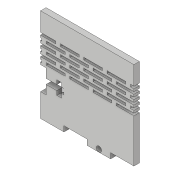
# Autodesk Inventor part: side2+hinge
Saved by Autodesk Inventor 2017 (Build 210142000, 142)
## iProperties
Created: 2019-05-21
Part Number: side2+hinge
Material: Generic
Document SubType Name: Modeling
Designer: markg
Density: 1 g/cm^3
Appearance: Default
Author: markg
Autodesk Inventor part; units mm, degrees
ref_plane "YZ Plane" through (0, 0, 0) normal (1, 0, 0) x (0, 1, 0)
ref_plane "XZ Plane" through (0, 0, 0) normal (0, 1, 0) x (-1, 0, 0)
ref_plane "XY Plane" through (0, 0, 0) normal (0, 0, 1) x (1, 0, 0)
sketch "Sketch1" plane through (0, 0, 0) normal (0, 0, 1) x (1, 0, 0)
  line L0 (-25.4, -25.4) -> (25.4, -25.4)
  line L1 (25.4, -25.4) -> (25.4, 25.4)
  line L2 (25.4, 25.4) -> (-25.4, 25.4)
  line L3 (-25.4, 25.4) -> (-25.4, -25.4)
  line L4 (-25.4, -25.4) -> (25.4, 25.4) construction
  line L5 (25.4, -25.4) -> (-25.4, 25.4) construction
  point P0 (0, 0)
  dimension "d0" = 50.8
  dimension "d1" = 50.8
  constraints: 12 end point, 2 midpoint, 2 parallel, 1 horizontal, 1 perpendicular
  measures "d0" distance of L2.end L1.end
  measures "d1" distance of L1.end L0.end
extrude "Extrusion1" add sketch "Sketch1" along normal blind 2.9718
sketch "Sketch2" plane through (0, 0, 2.9718) normal (0, 0, 1) x (1, 0, 0)
  line L0 (-25.4, -25.4) -> (25.4, -25.4) projected
  line L1 (25.4, -25.4) -> (12.7, -25.4)
  line L2 (12.7, -25.4) -> (12.7, -22.4282)
  line L3 (12.7, -22.4282) -> (25.4, -22.4282)
  line L4 (25.4, -22.4282) -> (25.4, -25.4)
  line L5 (0, -25.4) -> (-12.7, -25.4)
  line L6 (-12.7, -25.4) -> (-12.7, -22.4282)
  line L7 (-12.7, -22.4282) -> (0, -22.4282)
  line L8 (0, -22.4282) -> (0, -25.4)
  line L9 (-25.4, -12.7) -> (-22.4282, -12.7)
  line L10 (-22.4282, -12.7) -> (-22.4282, 0)
  line L11 (-22.4282, 0) -> (-25.4, 0)
  line L12 (-25.4, 0) -> (-25.4, -12.7)
  point P0 (0, 0)
  dimension "d4" = 12.7
  dimension "d5" = 2.9718
  dimension "d6" = 12.7
  dimension "d7" = 2.9718
  dimension "d8" = 2.9718
  dimension "d9" = 12.7
  dimension "d10" = 12.7
  constraints: 24 end point, 6 parallel, 3 horizontal, 3 perpendicular, 1 midpoint
  measures "d4" distance of L2.end L3.end
  measures "d5" distance of L1.end L2.end
  measures "d6" distance of L6.end L7.end
  measures "d7" distance of L5.end L6.end
  measures "d8" distance of L11.end L10.end
  measures "d9" distance of L10.end L9.end
  measures "d10" distance between parallel lines of L0 L9
extrude "Extrusion2" cut sketch "Sketch2" against normal blind 2.9718
sketch "Sketch3" plane through (0, 0, 0) normal (0, 0, -1) x (-1, 0, 0)
  line L0 (-26.035, 1.27) -> (-15.875, 1.27)
  line L1 (-15.875, 1.27) -> (-15.875, 2.54)
  line L2 (-15.875, 2.54) -> (-26.035, 2.54)
  line L3 (-26.035, 2.54) -> (-26.035, 1.27)
  line L4 (-25.4, -22.4282) -> (-25.4, 25.4) projected
  line L5 (-20.955, 3.81) -> (-10.795, 3.81)
  line L6 (-10.795, 3.81) -> (-10.795, 5.08)
  line L7 (-10.795, 5.08) -> (-20.955, 5.08)
  line L8 (-20.955, 5.08) -> (-20.955, 3.81)
  line L9 (-33.655, 3.81) -> (-23.495, 3.81)
  line L10 (-23.495, 3.81) -> (-23.495, 5.08)
  line L11 (-23.495, 5.08) -> (-33.655, 5.08)
  line L12 (-33.655, 5.08) -> (-33.655, 3.81)
  line L13 (-13.335, 1.27) -> (-3.175, 1.27)
  line L14 (-3.175, 1.27) -> (-3.175, 2.54)
  line L15 (-3.175, 2.54) -> (-13.335, 2.54)
  line L16 (-13.335, 2.54) -> (-13.335, 1.27)
  line L17 (9.525, 1.27) -> (9.525, 2.54)
  line L18 (4.445, 3.81) -> (14.605, 3.81)
  line L19 (14.605, 5.08) -> (4.445, 5.08)
  line L20 (4.445, 5.08) -> (4.445, 3.81)
  line L21 (-0.635, 1.27) -> (9.525, 1.27)
  line L22 (9.525, 2.54) -> (-0.635, 2.54)
  line L23 (-0.635, 2.54) -> (-0.635, 1.27)
  line L24 (12.065, 2.54) -> (12.065, 1.27)
  line L25 (14.605, 3.81) -> (14.605, 5.08)
  line L26 (22.225, 2.54) -> (12.065, 2.54)
  line L27 (12.065, 1.27) -> (22.225, 1.27)
  line L28 (22.225, 1.27) -> (22.225, 2.54)
  line L29 (1.905, 3.81) -> (1.905, 5.08)
  line L30 (1.905, 5.08) -> (-8.255, 5.08)
  line L31 (-8.255, 5.08) -> (-8.255, 3.81)
  line L32 (-8.255, 3.81) -> (1.905, 3.81)
  line L33 (34.925, 1.27) -> (34.925, 2.54)
  line L34 (29.845, 3.81) -> (40.005, 3.81)
  line L35 (40.005, 5.08) -> (29.845, 5.08)
  line L36 (29.845, 5.08) -> (29.845, 3.81)
  line L37 (24.765, 1.27) -> (34.925, 1.27)
  line L38 (34.925, 2.54) -> (24.765, 2.54)
  line L39 (24.765, 2.54) -> (24.765, 1.27)
  line L40 (37.465, 2.54) -> (37.465, 1.27)
  line L41 (40.005, 3.81) -> (40.005, 5.08)
  line L42 (47.625, 2.54) -> (37.465, 2.54)
  line L43 (37.465, 1.27) -> (47.625, 1.27)
  line L44 (47.625, 1.27) -> (47.625, 2.54)
  line L45 (27.305, 3.81) -> (27.305, 5.08)
  line L46 (27.305, 5.08) -> (17.145, 5.08)
  line L47 (17.145, 5.08) -> (17.145, 3.81)
  line L48 (17.145, 3.81) -> (27.305, 3.81)
  line L49 (-15.875, 6.35) -> (-15.875, 7.62)
  line L50 (-20.955, 8.89) -> (-10.795, 8.89)
  line L51 (-10.795, 10.16) -> (-20.955, 10.16)
  line L52 (-20.955, 10.16) -> (-20.955, 8.89)
  line L53 (-26.035, 6.35) -> (-15.875, 6.35)
  line L54 (-15.875, 7.62) -> (-26.035, 7.62)
  line L55 (-26.035, 7.62) -> (-26.035, 6.35)
  line L56 (-13.335, 7.62) -> (-13.335, 6.35)
  line L57 (-10.795, 8.89) -> (-10.795, 10.16)
  line L58 (-3.175, 7.62) -> (-13.335, 7.62)
  line L59 (-13.335, 6.35) -> (-3.175, 6.35)
  line L60 (-3.175, 6.35) -> (-3.175, 7.62)
  line L61 (-23.495, 8.89) -> (-23.495, 10.16)
  line L62 (-23.495, 10.16) -> (-33.655, 10.16)
  line L63 (-33.655, 10.16) -> (-33.655, 8.89)
  line L64 (-33.655, 8.89) -> (-23.495, 8.89)
  line L65 (9.525, 6.35) -> (9.525, 7.62)
  line L66 (4.445, 8.89) -> (14.605, 8.89)
  line L67 (14.605, 10.16) -> (4.445, 10.16)
  line L68 (4.445, 10.16) -> (4.445, 8.89)
  line L69 (-0.635, 6.35) -> (9.525, 6.35)
  line L70 (9.525, 7.62) -> (-0.635, 7.62)
  line L71 (-0.635, 7.62) -> (-0.635, 6.35)
  line L72 (12.065, 7.62) -> (12.065, 6.35)
  line L73 (14.605, 8.89) -> (14.605, 10.16)
  line L74 (22.225, 7.62) -> (12.065, 7.62)
  line L75 (12.065, 6.35) -> (22.225, 6.35)
  line L76 (22.225, 6.35) -> (22.225, 7.62)
  line L77 (1.905, 8.89) -> (1.905, 10.16)
  line L78 (1.905, 10.16) -> (-8.255, 10.16)
  line L79 (-8.255, 10.16) -> (-8.255, 8.89)
  line L80 (-8.255, 8.89) -> (1.905, 8.89)
  line L81 (34.925, 6.35) -> (34.925, 7.62)
  line L82 (29.845, 8.89) -> (40.005, 8.89)
  line L83 (40.005, 10.16) -> (29.845, 10.16)
  line L84 (29.845, 10.16) -> (29.845, 8.89)
  line L85 (24.765, 6.35) -> (34.925, 6.35)
  line L86 (34.925, 7.62) -> (24.765, 7.62)
  line L87 (24.765, 7.62) -> (24.765, 6.35)
  line L88 (37.465, 7.62) -> (37.465, 6.35)
  line L89 (40.005, 8.89) -> (40.005, 10.16)
  line L90 (47.625, 7.62) -> (37.465, 7.62)
  line L91 (37.465, 6.35) -> (47.625, 6.35)
  line L92 (47.625, 6.35) -> (47.625, 7.62)
  line L93 (27.305, 8.89) -> (27.305, 10.16)
  line L94 (27.305, 10.16) -> (17.145, 10.16)
  line L95 (17.145, 10.16) -> (17.145, 8.89)
  line L96 (17.145, 8.89) -> (27.305, 8.89)
  line L97 (-15.875, 11.43) -> (-15.875, 12.7)
  line L98 (-20.955, 13.97) -> (-10.795, 13.97)
  line L99 (-10.795, 15.24) -> (-20.955, 15.24)
  line L100 (-20.955, 15.24) -> (-20.955, 13.97)
  line L101 (-26.035, 11.43) -> (-15.875, 11.43)
  line L102 (-15.875, 12.7) -> (-26.035, 12.7)
  line L103 (-26.035, 12.7) -> (-26.035, 11.43)
  line L104 (-13.335, 12.7) -> (-13.335, 11.43)
  line L105 (-10.795, 13.97) -> (-10.795, 15.24)
  line L106 (-3.175, 12.7) -> (-13.335, 12.7)
  line L107 (-13.335, 11.43) -> (-3.175, 11.43)
  line L108 (-3.175, 11.43) -> (-3.175, 12.7)
  line L109 (-23.495, 13.97) -> (-23.495, 15.24)
  line L110 (-23.495, 15.24) -> (-33.655, 15.24)
  line L111 (-33.655, 15.24) -> (-33.655, 13.97)
  line L112 (-33.655, 13.97) -> (-23.495, 13.97)
  line L113 (9.525, 11.43) -> (9.525, 12.7)
  line L114 (4.445, 13.97) -> (14.605, 13.97)
  line L115 (14.605, 15.24) -> (4.445, 15.24)
  line L116 (4.445, 15.24) -> (4.445, 13.97)
  line L117 (-0.635, 11.43) -> (9.525, 11.43)
  line L118 (9.525, 12.7) -> (-0.635, 12.7)
  line L119 (-0.635, 12.7) -> (-0.635, 11.43)
  line L120 (12.065, 12.7) -> (12.065, 11.43)
  line L121 (14.605, 13.97) -> (14.605, 15.24)
  line L122 (22.225, 12.7) -> (12.065, 12.7)
  line L123 (12.065, 11.43) -> (22.225, 11.43)
  line L124 (22.225, 11.43) -> (22.225, 12.7)
  line L125 (1.905, 13.97) -> (1.905, 15.24)
  line L126 (1.905, 15.24) -> (-8.255, 15.24)
  line L127 (-8.255, 15.24) -> (-8.255, 13.97)
  line L128 (-8.255, 13.97) -> (1.905, 13.97)
  line L129 (34.925, 11.43) -> (34.925, 12.7)
  line L130 (29.845, 13.97) -> (40.005, 13.97)
  line L131 (40.005, 15.24) -> (29.845, 15.24)
  line L132 (29.845, 15.24) -> (29.845, 13.97)
  line L133 (24.765, 11.43) -> (34.925, 11.43)
  line L134 (34.925, 12.7) -> (24.765, 12.7)
  line L135 (24.765, 12.7) -> (24.765, 11.43)
  line L136 (37.465, 12.7) -> (37.465, 11.43)
  line L137 (40.005, 13.97) -> (40.005, 15.24)
  line L138 (47.625, 12.7) -> (37.465, 12.7)
  line L139 (37.465, 11.43) -> (47.625, 11.43)
  line L140 (47.625, 11.43) -> (47.625, 12.7)
  line L141 (27.305, 13.97) -> (27.305, 15.24)
  line L142 (27.305, 15.24) -> (17.145, 15.24)
  line L143 (17.145, 15.24) -> (17.145, 13.97)
  line L144 (17.145, 13.97) -> (27.305, 13.97)
  point P0 (0, 0)
  point P1 (25.4, 0)
  point P2 (50.8, 0)
  point P3 (0, 5.08)
  point P4 (25.4, 5.08)
  point P5 (50.8, 5.08)
  point P6 (0, 10.16)
  point P7 (25.4, 10.16)
  point P8 (50.8, 10.16)
  dimension "d14" = 1.27
  dimension "d15" = 10.16
  dimension "d16" = 1.27
  dimension "d17" = 10.16
  dimension "d18" = 1.27
  dimension "d19" = 1.27
  dimension "d20" = 10.16
  dimension "d21" = 1.27
  dimension "d22" = 5.08
  dimension "d23" = 2.54
  dimension "d24" = 1.27
  dimension "d25" = 1.27
  dimension "d26" = 10.16
  dimension "d27" = 0
  dimension "d28" = 2.54
  dimension "d31" = 25.4
  dimension "d34" = 5.08
  dimension "d37" = 26.035
  constraints: 288 end point, 8 parallel, 5 horizontal, 4 perpendicular, 2 collinear, 1 vertical, 262 other
  measures "d14" distance of L0.end L1.end
  measures "d15" distance of L1.end L2.end
  measures "d16" distance of L5.end L6.end
  measures "d17" distance of L6.end L7.end
  measures "d18" distance between parallel lines of L2 L5
  measures "d19" distance of L9.end L10.end
  measures "d20" distance of L10.end L11.end
  measures "d21" distance between parallel lines of L2 L9
  measures "d22" distance between parallel lines of L3 L8
  measures "d23" distance between parallel lines of L8 L10
  measures "d24" distance from line of point (0, 0) L0
  measures "d25" distance of L14.start L14.end
  measures "d26" distance of L14.end L15.end
  measures "d27" distance between parallel lines of L13 L0
  measures "d28" distance between parallel lines of L1 L16
  measures "d31" distance of L1.end L17.end
  measures "d34" distance of L1.end L49.end
  measures "d37" distance from line of L3 point (0, 0)
extrude "Extrusion4" cut sketch "Sketch3" against normal blind 2.9718 contours L3 L2 L4 L0 | L112 L111 L110 L4 | L4 L110 L109 L112 | L101 L103 L102 L4 | L4 L102 L97 L101 | L64 L63 L62 L4 | L4 L62 L61 L64 | L53 L55 L54 L4 | L4 L54 L49 L53 | L9 L12 L11 L4 | L4 L11 L10 L9 | L4 L2 L1 L0 | L8 L7 L6 L5 | L16 L15 L14 L13 | L21 L23 L22 L17 | L20 L19 L25 L18 | L26 L28 L27 L24 | L32 L31 L30 L29 | L37 L39 L38 L33 | L48 L47 L46 L45 | L52 L51 L57 L50 | L58 L60 L59 L56 | L69 L71 L70 L65 | L68 L67 L73 L66 | L74 L76 L75 L72 | L80 L79 L78 L77 | L85 L87 L86 L81 | L96 L95 L94 L93 | L100 L99 L105 L98 | L106 L108 L107 L104 | L117 L119 L118 L113 | L116 L115 L121 L114 | L122 L124 L123 L120 | L128 L127 L126 L125 | L133 L135 L134 L129 | L144 L143 L142 L141
sketch "Sketch4" plane through (0, 0, 0) normal (0, 0, -1) x (-1, 0, 0)
  circle A0 centre (-6.35, -23.9141) radius 1.4351
  line L0 (0, -25.4) -> (0, -22.4282) projected
  line L1 (0, -25.4) -> (-12.7, -25.4) projected
  line L2 (25.4, -25.4) -> (12.7, -25.4) projected
  line L3 (12.7, -22.4282) -> (12.7, -25.4) projected
  point P0 (0, 0)
  dimension "d43" = 2.8702
  dimension "d44" = 6.35
  dimension "d45" = 1.4859
  constraints: 1 centre point
  measures "d43" diameter of A0
  measures "d44" distance from line of A0.centre L0
  measures "d45" distance from line of L1 A0.centre
extrude "Extrusion6" cut sketch "Sketch4" against normal blind 2.9718
sketch "Sketch5" plane through (0, 0, 0) normal (0, 0, -1) x (-1, 0, 0)
  line L0 (22.4282, -4.9657) -> (16.5862, -4.9657)
  line L1 (16.5862, -4.9657) -> (16.5862, -2.7305)
  line L2 (16.5862, -2.7305) -> (14.0462, -2.7305)
  line L3 (14.0462, -2.7305) -> (14.0462, -4.9657)
  line L4 (14.0462, -4.9657) -> (12.7, -4.9657)
  line L5 (12.7, -4.9657) -> (12.7, -7.8359)
  line L6 (12.7, -7.8359) -> (14.0462, -7.8359)
  line L7 (14.0462, -7.8359) -> (14.0462, -10.0711)
  line L8 (14.0462, -10.0711) -> (16.5862, -10.0711)
  line L9 (16.5862, -10.0711) -> (16.5862, -7.8359)
  line L10 (16.5862, -7.8359) -> (22.4282, -7.8359)
  line L11 (22.4282, 0) -> (22.4282, -12.7) projected
  line L12 (22.4282, -4.9657) -> (22.4282, -7.8359)
  line L13 (25.4, -12.7) -> (22.4282, -12.7) projected
  point P0 (0, 0)
  dimension "d52" = 5.842
  dimension "d53" = 1.3462
  dimension "d54" = 2.54
  dimension "d55" = 2.54
  dimension "d56" = 2.8702
  dimension "d57" = 2.8702
  dimension "d58" = 2.2352
  dimension "d59" = 2.2352
  dimension "d60" = 2.2352
  dimension "d61" = 4.8641
  constraints: 24 end point, 9 perpendicular, 3 point on line, 1 horizontal, 1 vertical
  measures "d52" distance of L0.start L0.end
  measures "d53" distance of L3.end L4.end
  measures "d54" distance of L1.end L2.end
  measures "d55" distance of L7.end L8.end
  measures "d56" distance of L4.end L5.end
  measures "d57" distance between parallel lines of L10 L0
  measures "d58" distance of L0.end L1.end
  measures "d59" distance of L8.end L9.end
  measures "d60" distance of L2.end L3.end
  measures "d61" distance between parallel lines of L10 L13
extrude "Extrusion7" cut sketch "Sketch5" against normal blind 2.9718
body "Solid1"
